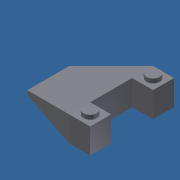
# Autodesk Inventor part: LEGO Brick 4858
Saved by Autodesk Inventor 2011 SP2 (Build 150309200, 309)
## iProperties
Created: 2011-09-27
Part Number: LEGO Brick 4858
Cost Center: 0 kg
Material: Steel
Document SubType Name: Modeling
Designer: BvH
Authority: 0 mm^3
Stock Number: =<Filenr>_<Document number>
Density: 7.85 g/cm^3
Company: Allseas Engineering BV
Subject: =<Title><TITLE 1_2> <TITLE 2_2>
Author: BvH
Act. Code: DW000
SaveDate: 2011-07-28
SaveTime: 18:32
FileName: Standard
TotalMass: 0 kg
TotalVolume: 0 mm^3
Autodesk Inventor part; units mm, degrees
ref_plane "YZ Plane" through (0, 0, 0) normal (1, 0, 0) x (0, 1, 0)
ref_plane "XZ Plane" through (0, 0, 0) normal (0, 1, 0) x (-1, 0, 0)
ref_plane "XY Plane" through (0, 0, 0) normal (0, 0, 1) x (1, 0, 0)
sketch "Sketch1" plane through (0, 0, 0) normal (0, 0, 1) x (1, 0, 0)
  line L0 (-22.4, 0) -> (22.4, 0) construction
  line L1 (0, -22.4) -> (0, 22.4) construction
  line L2 (-16, 16) -> (16, 16)
  line L3 (16, 16) -> (16, -16)
  line L4 (16, -16) -> (-16, -16)
  line L5 (-16, -16) -> (-16, 16)
  line L6 (8, 16) -> (-16, 8)
  line L7 (-16, -8) -> (8, -16)
  line L8 (16, 8) -> (8, 8)
  line L9 (8, 8) -> (8, -8)
  line L10 (8, -8) -> (16, -8)
  point P0 (-16, 0)
  point P1 (0, 16)
  point P2 (8, 0)
  dimension "d0" = 32
  dimension "d1" = 32
  dimension "d5" = 16
  dimension "d9" = 8
  dimension "d10" = 16
  constraints: 18 end point, 11 point on line, 4 horizontal, 3 midpoint, 3 vertical, 1 equal length
  measures "d0" distance between parallel lines of L3 L5
  measures "d1" distance between parallel lines of L4 L2
  measures "d5" distance of L7.start L6.end
  measures "d9" distance between parallel lines of L3 L9
  measures "d10" distance between parallel lines of L10 L8
extrude "Extrusion1" add sketch "Sketch1" along normal blind 9.6 contours L2 L3 L8 L9 L10 L4 L7 L5 L6 | L3 L10 L9 L8
sketch "Sketch2" plane through (0, 0, 0) normal (0, 1, 0) x (-1, 0, 0)
  line L0 (-16, 0) -> (-16, 9.6) projected
  line L1 (-16, 9.6) -> (-8, 9.6) projected
  line L2 (16, 0) -> (16, 9.6) projected
  line L3 (16, 0) -> (-16, 0)
  line L4 (-8, 9.6) -> (16, 1.6)
  dimension "d6" = 1.6
  constraints: 4 end point, 1 horizontal, 1 point on line
  measures "d6" distance from line of L3 L4.end
extrude "Extrusion2" cut sketch "Sketch2" along normal through all both and the other way through all keep common part
extrude "Extrusion4" cut sketch "Sketch1" along normal through all both and the other way through all contours L3 L10 L9 L8
shell "Shell1" thickness 0.8 removed faces 1 at (-8, 2.6667, 0)
sketch "Sketch3" plane through (0, 0, 9.6) normal (0, 0, 1) x (1, 0, 0)
  line L0 (16, 16) -> (16, -16) construction
  line L1 (-22.4, 0) -> (22.4, 0) construction
  line L2 (12, 12) -> (12, -12) construction
  circle A0 centre (12, 12) radius 2.5
  circle A1 centre (12, -12) radius 2.5
  point P0 (12, 0)
  dimension "d11" = 4
  dimension "d12" = 24
  dimension "d13" = 5
  constraints: 2 centre point, 2 coincident, 2 end point, 1 equal radius, 1 midpoint, 1 point on line, 1 vertical
  measures "d11" distance between parallel lines of L0 L2
  measures "d12" distance of L2.start L2.end
  measures "d13" diameter of A0
extrude "Extrusion3" add sketch "Sketch3" along normal blind 1.6
body "Solid1"
